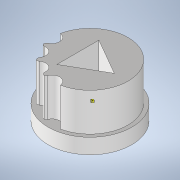
# Autodesk Inventor part: handle_base2
Saved by Autodesk Inventor 2021 (Build 250183000, 183)
## iProperties
Created: 2021-06-02
Part Number: handle_base2
Material: Generic
Document SubType Name: Modeling
Designer: teh18
Density: 1 g/cm^3
Appearance: Default
Author: teh18
Autodesk Inventor part; units mm, degrees
ref_plane "YZ Plane" through (0, 0, 0) normal (1, 0, 0) x (0, 1, 0)
ref_plane "XZ Plane" through (0, 0, 0) normal (0, 1, 0) x (-1, 0, 0)
sketch "Sketch1" plane through (0, 0, 0) normal (0, 0, 1) x (1, 0, 0)
  circle A0 centre (0, 0) radius 27.5 projected
  circle A1 centre (0, 0) radius 35
  line L0 (16, 0) -> (-8, -13.8564)
  line L1 (-8, 13.8564) -> (16, 0)
  line L2 (-8, -13.8564) -> (-8, 13.8564)
  circle A2 centre (0, 0) radius 25
  circle A3 centre (-25, 0) radius 5
  circle A4 centre (-21.6506, 12.5) radius 5
  circle A5 centre (-12.5, 21.6506) radius 5
  circle A6 centre (0, 25) radius 5
  circle A7 centre (0, 0) radius 38 projected
  point P0 (4.9749, 24.5)
  point P1 (-4.9749, 24.5)
  point P2 (-7.9416, 23.7051)
  point P3 (-16.5584, 18.7302)
  point P4 (-18.7302, 16.5584)
  point P5 (-23.7051, 7.9416)
  point P6 (-24.5, 4.9749)
  point P7 (-24.5, -4.9749)
  dimension "d5" = 70
  dimension "d14" = 10
  dimension "d15" = 10
  dimension "d18" = 90
  constraints: 6 end point, 5 centre point, 1 coincident, 1 vertical, 15 other
  measures "d5" diameter of A1
  measures "d15" diameter of A3
ref_plane "Work Plane7" through (-38, -38, 25) normal (0, 0, -1) x (0, 1, 0)
extrude "Extrusion1" add sketch "Sketch1" along normal up to surface (25 mm away) contours A3 A2 A4 A5 A6
fillet "Fillet1" radius 2 6 edges at (-24.5, 4.9749, 12.5) (-23.7051, 7.9416, 12.5) (-18.7302, 16.5584, 12.5) (-16.5584, 18.7302, 12.5) (-7.9416, 23.7051, 12.5) (-4.9749, 24.5, 12.5)
sketch "Sketch3" plane through (0, 0, 25) normal (0, 0, 1) x (0, 1, 0)
  circle A0 centre (0, 0) radius 28 projected
  circle A1 centre (0, 0) radius 6
  circle A2 centre (0, 0) radius 27.5
  dimension "d13" = 0.5
  constraints: 2 centre point, 2 other
  measures "d13" radial gap between concentric circles of A0 A2
extrude "Extrusion3" add sketch "Sketch3" along normal blind 10 contours A2
body "Solid1"
